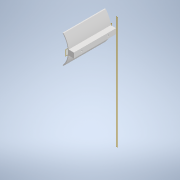
# Autodesk Inventor part: LegSupport
Saved by Autodesk Inventor 2022 (Build 260153000, 153)
## iProperties
Created: 2022-02-23
Part Number: LegSupport
Material: Generic
Document SubType Name: Modeling
Designer: siwat
Density: 1 g/cm^3
Appearance: Default
Author: siwat
Autodesk Inventor part; units mm, degrees
ref_plane "YZ Plane" through (0, 0, 0) normal (1, 0, 0) x (0, 1, 0)
ref_plane "XZ Plane" through (0, 0, 0) normal (0, 1, 0) x (-1, 0, 0)
ref_plane "XY Plane" through (0, 0, 0) normal (0, 0, 1) x (1, 0, 0)
ref_plane "Work Plane1" through (-14.5039, 0, 0) normal (0, 0, 1) x (1, 0, 0)
sketch "Sketch1" plane through (-14.5039, 0, 0) normal (0, 0, 1) x (1, 0, 0)
  line L0 (-0.3057, 380.2711) -> (-25.3057, 380.2711)
  line L1 (-25.3057, 380.2711) -> (-25.3057, 360.2711)
  line L2 (-25.3057, 360.2711) -> (-0.3057, 360.2711)
  line L3 (-0.3057, 360.2711) -> (-0.3057, 380.2711)
  arc A0 (-40.5531, 315.2711) -> (-40.5531, 425.2711) centre (-105.3057, 370.2711) ccw
  line L4 (-40.5531, 425.2711) -> (-40.5531, 315.2711) construction
  line L5 (-40.5531, 425.2711) -> (69.4469, 425.2711) construction
  line L6 (-40.5531, 315.2711) -> (-44.5531, 315.2711)
  line L7 (-40.5531, 425.2711) -> (-44.5531, 425.2711)
  arc A1 (-44.5531, 315.2711) -> (-44.5531, 425.2711) centre (-105.3057, 370.2711) ccw
  point P0 (14.5039, 0)
  point P1 (-20.938, 380.2711)
  point P2 (-20.938, 360.2711)
  dimension "d0" = 25
  dimension "d1" = 20
  dimension "d2" = 110
  dimension "d3" = 90
  dimension "d4" = 45
  dimension "d5" = 105
  dimension "d6" = 4
  constraints: 16 end point, 4 point on circle, 3 horizontal, 2 centre point, 2 parallel, 2 perpendicular, 1 concentric, 1 point on line
  measures "d0" distance of L2.end L1.end
  measures "d1" distance of L1.end L0.end
  measures "d2" distance of L4.start L4.end
  measures "d3" angle of L4 L5
  measures "d4" distance from line of L0 L4.start
  measures "d5" distance from line of A0.centre L3
  measures "d6" distance of L4.end L6.end
extrude "Extrusion1" add sketch "Sketch1" along normal blind 165 contours L3 L2 A0 L0 | A0 L2 A1 L0 | L0 A1 L7 A0 | A0 L6 A1 L2
sketch "Sketch2" plane through (-14.8095, 360.2711, 0) normal (1, 0, 0) x (0, 0, -1)
  circle A0 centre (-30, 10) radius 2.75
  circle A1 centre (-135, 10) radius 2.75
  line L0 (-165, 0) -> (-165, 20) projected
  line L1 (0, 0) -> (0, -45) projected
  line L2 (-30, 10) -> (-135, 10)
  line L3 (0, -45) -> (-165, -45) projected
  point P0 (0, -360.2711)
  dimension "d10" = 5.5
  dimension "d11" = 5.5
  dimension "d12" = 30
  dimension "d13" = 30
  dimension "d17" = 55
  constraints: 2 centre point, 2 end point, 1 horizontal
  measures "d10" diameter of A0
  measures "d11" diameter of A1
  measures "d12" distance from line of L0 L2.end
  measures "d13" distance from line of L1 L2.start
  measures "d17" distance between parallel lines of L3 L2
extrude "Extrusion2" cut sketch "Sketch2" against normal through all
ref_plane "Work Plane2" through (-39.8095, 360.2711, 0) normal (1, 0, 0) x (0, 0, -1)
sketch "Sketch4" plane through (-39.8095, 360.2711, 0) normal (1, 0, 0) x (0, 0, -1)
  circle A0 centre (-30, 10) radius 2.75 projected
  circle A1 centre (-30, 10) radius 5.75
  circle A2 centre (-135, 10) radius 2.75 projected
  circle A3 centre (-135, 10) radius 5.75
  point P0 (0, -360.2711)
  dimension "d18" = 11.5
  dimension "d19" = 11.5
  constraints: 2 centre point, 2 coincident
  measures "d18" diameter of A1
  measures "d19" diameter of A3
extrude "Extrusion3" cut sketch "Sketch4" along normal blind 20 contours A0 | A1 | A3
equation "\"d4\" = -0.5 * d1 + 0.5 * d2"
body "Solid1"
